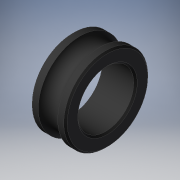
# Autodesk Inventor part: 040102DR-18-H8_ir
Saved by Autodesk Inventor 2024 (Build 280153000, 153)
## iProperties
Created: 2023-06-20
Part Number: 040102DR-18-H8_ir
Material: Generic
Catalog Web Link: www.cadenas.de
Description: DR-H ir-D-Series bearings
Vendor: TOKBEARING
Document SubType Name: Modeling
Designer: psAdmin
Manufacturer: TOKBEARING
Mass: 8700 g
Surface Area: 4.3226 cm^2
Volume: 0.254198 cm^3
Density: 1 g/cm^3
Appearance: PSOLRGB-175-175-175
Category: PARTsolutions
Company: TOKBEARING
PSOL_IDENT_0: {$CADENAS_DATA/23d-libs/tok_bearing/d_series_bearings/dr_h/dr_h_ir.prj},177 {VTYP=3D},{NB=040102DR-1
PSOL_IDENT_1: 8-H8_ir},{LINA=040102DR-18-H8_ir},{NN=DR-H ir},{DATE=16.12.2020 00:38:04},{GEOMDATE=19.02.2013 00:00
PSOL_IDENT_2: :00},{VERSION=},{LINEID=1710},{WBVAR=},{WBNUMERIC=}  {NB=040102DR-18-H8_ir},{LINA=040102DR-18-H8_ir}
PSOL_IDENT_3: ,{KT=DUMMY},{IDNR=},{CODE=040102},{PN=DR-18-H8},{D=18},{SD=8.0},{W=5.0},{W1=-},{W1X=0.000},{W2=-},{W
PSOL_IDENT_4: 2X=0.000},{LOAD=49 (5)},{TYPE=11},{QTY=3.000},{GW=8.7},{BD=3.2},{OP=42.704},{N=6},{R=6.8},{GP=1.4}
NB: 040102DR-18-H8_ir
NN: DR-H ir
NT: D-Series bearings
NBSYN: $CODE.$PN._ir
LINA: 040102DR-18-H8_ir
CATALOG: TOK, Inc
CODE: 040102
PN: DR-18-H8
D: 18
SD: 8
W: 5
W1: -
W2: -
LOAD: 49 (5)
TYPE: 11
QTY: 3.000
GW: 8.7
SUPPLIER: TOKBEARING
ARTICLENO: 040102DR-18-H8_ir
BOMINFO: 040102DR-18-H8_ir
CREATOR: CADENAS GmbH
Title: 040102DR-18-H8_ir
Author: Cadenas PARTsolutions
Comments: D-Series bearings
Autodesk Inventor part; units mm, degrees
sketch "Sketch_3" plane through (0, 0, 0) normal (0, 0, 1) x (1, 0, 0)
  line L0 (5, 0) -> (0, 0)
  line L1 (0, 4.25) -> (0.25, 4)
  line L2 (0.25, 4) -> (4.75, 4)
  line L3 (4.75, 4) -> (5, 4.25)
  line L4 (5, 4.25) -> (5, 5.75)
  line L5 (5, 5.75) -> (4.75, 6)
  line L6 (4.75, 6) -> (3.8856, 6)
  arc A0 (1.1144, 6) -> (3.8856, 6) centre (2.5, 6.8) ccw
  line L7 (1.1144, 6) -> (0.25, 6)
  line L8 (0.25, 6) -> (0, 5.75)
  line L9 (0, 5.75) -> (0, 4.25)
  constraints: 20 end point, 2 point on circle, 1 centre point
revolve "Revolution1" add sketch "Sketch_3" angle 360 about axis through (5, 0, 0) along (1, 0, 0)
ref_plane "Dummy_IR_XY" through (0, 0, 0) normal (1, 0, 0) x (0, 0, -1)
ref_plane "Dummy_IR_YZ" through (0, 0, 0) normal (0, 0, -1) x (0, 1, 0)
ref_plane "Dummy_IR_ZX" through (0, 0, 0) normal (0, 1, 0) x (1, 0, 0)
ref_plane "IR_OR_XY" through (0, 0, 0) normal (1, 0, 0) x (0, 0, -1)
ref_plane "IR_OR_YZ" through (0, 0, 0) normal (0, 0, -1) x (0, 1, 0)
ref_plane "IR_OR_ZX" through (0, 0, 0) normal (0, 1, 0) x (1, 0, 0)
body "Solid1"
